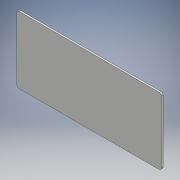
# Autodesk Inventor part: layer1
Saved by Autodesk Inventor 2017 (Build 210142000, 142)
## iProperties
Created: 2021-06-16
Part Number: layer1
Material: Generic
Document SubType Name: Modeling
Designer: Jack
Density: 1 g/cm^3
Appearance: Default
Author: Jack
Autodesk Inventor part; units mm, degrees
ref_plane "YZ Plane" through (0, 0, 0) normal (1, 0, 0) x (0, 1, 0)
ref_plane "XZ Plane" through (0, 0, 0) normal (0, 1, 0) x (-1, 0, 0)
ref_plane "XY Plane" through (0, 0, 0) normal (0, 0, 1) x (1, 0, 0)
sketch "Sketch1" plane through (0, 0, 0) normal (0, 1, 0) x (-1, 0, 0)
  line L0 (-163.4597, 74.0791) -> (-163.4597, -75.7459)
  line L1 (-158.4597, 79.0791) -> (177.1033, 79.0791)
  arc A0 (-158.4597, 79.0791) -> (-163.4597, 74.0791) centre (-158.4597, 74.0791) ccw
  arc A1 (-163.4597, -75.7459) -> (-158.4597, -80.7459) centre (-158.4597, -75.7459) ccw
  line L2 (182.1033, -75.7459) -> (182.1033, 74.0791)
  line L3 (177.1033, -80.7459) -> (-158.4597, -80.7459)
  arc A2 (177.1033, -80.7459) -> (182.1033, -75.7459) centre (177.1033, -75.7459) ccw
  arc A3 (182.1033, 74.0791) -> (177.1033, 79.0791) centre (177.1033, 74.0791) ccw
  point P0 (0, 0)
  constraints: 8 end point, 8 point on circle, 4 centre point
extrude "Extrusion1" add sketch "Sketch1" along normal blind 4
body "Solid1"
